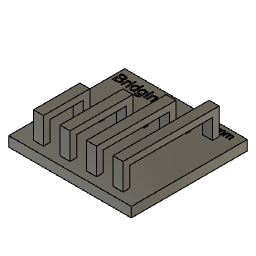
bridging (Autodesk Fusion 360 design; units mm, degrees)
Autodesk Fusion 360 part; units mm, degrees
sketch "Sketch1" plane through (0, 0, 0) normal (0, 0, 1) x (1, 0, 0)
  line L0 (0, 0) -> (37, 0)
  line L1 (37, 0) -> (37, 35)
  line L2 (37, 35) -> (0, 35)
  line L3 (0, 35) -> (0, 0)
  dimension "d1" = 35
  dimension "d2" = 37
  constraint horizontal L0
  constraint vertical L1
  constraint horizontal L2
  constraint vertical L3
  constraint coincident L0.start L3.end
  measures "d1" distance of L0.start L2.end
  measures "d2" distance of L0.start L0.end
extrude "Extrude1" add sketch "Sketch1" along normal blind 3
sketch "Sketch2" plane through (0, 0, 3) normal (0, 0, 1) x (-1, 0, 0)
  line L0 (0, -35) -> (0, 0)
  line L1 (0, 0) -> (-37, 0)
  line L2 (-37, 0) -> (-37, -35)
  line L3 (-37, -35) -> (0, -35)
  line L4 (-5, -2.5) -> (-8, -2.5)
  line L5 (-8, -2.5) -> (-8, -4.5)
  line L6 (-8, -4.5) -> (-5, -4.5)
  line L7 (-5, -4.5) -> (-5, -2.5)
  line L8 (-13, -2.5) -> (-16, -2.5)
  line L9 (-16, -2.5) -> (-16, -4.5)
  line L10 (-13, -4.5) -> (-13, -2.5)
  line L11 (-16, -4.5) -> (-13, -4.5)
  line L12 (-21, -2.5) -> (-24, -2.5)
  line L13 (-24, -2.5) -> (-24, -4.5)
  line L14 (-21, -4.5) -> (-21, -2.5)
  line L15 (-24, -4.5) -> (-21, -4.5)
  line L16 (-29, -2.5) -> (-32, -2.5)
  line L17 (-32, -2.5) -> (-32, -4.5)
  line L18 (-29, -4.5) -> (-29, -2.5)
  line L19 (-32, -4.5) -> (-29, -4.5)
  line L20 (-5, -14.5) -> (-8, -14.5)
  line L21 (-8, -14.5) -> (-8, -16.5)
  line L22 (-5, -16.5) -> (-5, -14.5)
  line L23 (-8, -16.5) -> (-5, -16.5)
  line L24 (-13, -19.5) -> (-16, -19.5)
  line L25 (-16, -19.5) -> (-16, -21.5)
  line L26 (-13, -21.5) -> (-13, -19.5)
  line L27 (-16, -21.5) -> (-13, -21.5)
  line L28 (-21, -24.5) -> (-24, -24.5)
  line L29 (-24, -24.5) -> (-24, -26.5)
  line L30 (-21, -26.5) -> (-21, -24.5)
  line L31 (-24, -26.5) -> (-21, -26.5)
  line L32 (-29, -29.5) -> (-32, -29.5)
  line L33 (-32, -29.5) -> (-32, -31.5)
  line L34 (-29, -31.5) -> (-29, -29.5)
  line L35 (-32, -31.5) -> (-29, -31.5)
  dimension "d5" = 3
  dimension "d6" = 2
  dimension "d7" = 5
  dimension "d8" = 2.5
  dimension "d9" = 3
  dimension "d10" = 2
  dimension "d11" = 3
  dimension "d12" = 2
  dimension "d13" = 3
  dimension "d14" = 2
  dimension "d15" = 3
  dimension "d16" = 2
  dimension "d17" = 3
  dimension "d18" = 2
  dimension "d19" = 3
  dimension "d20" = 2
  dimension "d21" = 3
  dimension "d22" = 2
  dimension "d23" = 10
  dimension "d24" = 15
  dimension "d25" = 20
  dimension "d26" = 25
  constraint horizontal L4
  constraint vertical L5
  constraint horizontal L6
  constraint vertical L7
  constraint horizontal L8
  constraint vertical L9
  constraint horizontal L11
  constraint vertical L10
  constraint horizontal L12
  constraint vertical L13
  constraint horizontal L15
  constraint vertical L14
  constraint horizontal L16
  constraint vertical L17
  constraint horizontal L19
  constraint vertical L18
  constraint horizontal L20
  constraint vertical L21
  constraint horizontal L23
  constraint vertical L22
  constraint horizontal L24
  constraint vertical L25
  constraint horizontal L27
  constraint vertical L26
  constraint horizontal L28
  constraint vertical L29
  constraint horizontal L31
  constraint vertical L30
  constraint horizontal L32
  constraint vertical L33
  constraint horizontal L35
  constraint vertical L34
  measures "d5" distance of L5 L7
  measures "d6" distance of L4 L6
  measures "d7" distance of L0 L7
  measures "d8" distance of L1 L4
  measures "d9" distance of L9 L10
  measures "d10" distance of L8 L11
  measures "d11" distance of L13 L14
  measures "d12" distance of L12 L15
  measures "d13" distance of L17 L18
  measures "d14" distance of L16 L19
  measures "d15" distance of L21 L22
  measures "d16" distance of L20 L23
  measures "d17" distance of L25 L26
  measures "d18" distance of L24 L27
  measures "d19" distance of L29 L30
  measures "d20" distance of L28 L31
  measures "d21" distance of L33 L34
  measures "d22" distance of L32 L35
  measures "d23" distance of L6 L20
  measures "d24" distance of L11 L24
  measures "d25" distance of L15 L28
  measures "d26" distance of L19 L32
extrude "Extrude2" add sketch "Sketch2" along normal blind 8 contours L4 L5 L6 L7 | L8 L9 L10 L11 | L12 L13 L14 L15 | L16 L17 L18 L19 | L20 L21 L22 L23 | L24 L25 L26 L27 | L28 L29 L30 L31 | L32 L33 L34 L35
sketch "Sketch3" plane through (0, 14.5, 0) normal (0, -1, 0) x (1, 0, 0)
  line L0 (5, 3) -> (8, 3)
  line L1 (8, 3) -> (8, 11)
  line L2 (8, 11) -> (5, 11)
  line L3 (5, 11) -> (5, 3)
  line L4 (5, 11) -> (8, 11)
  line L5 (8, 11) -> (8, 9)
  line L6 (8, 9) -> (5, 9)
  line L7 (5, 9) -> (5, 11)
  dimension "d29" = 2
  constraint horizontal L4
  constraint vertical L5
  constraint horizontal L6
  constraint vertical L7
  constraint coincident L2.end L3.start
  measures "d29" distance of L2.end L6.end
extrude "Extrude3" add sketch "Sketch3" along normal blind 10 contours L1 L2 L3 L4 L5 L6 L7
sketch "Sketch4" plane through (0, 19.5, 0) normal (0, -1, 0) x (1, 0, 0)
  line L0 (13, 3) -> (16, 3)
  line L1 (16, 3) -> (16, 11)
  line L2 (16, 11) -> (13, 11)
  line L3 (13, 11) -> (13, 3)
  line L4 (13, 11) -> (16, 11)
  line L5 (16, 11) -> (16, 9)
  line L6 (16, 9) -> (13, 9)
  line L7 (13, 9) -> (13, 11)
  dimension "d32" = 2
  constraint horizontal L4
  constraint vertical L5
  constraint horizontal L6
  constraint vertical L7
  constraint coincident L1 L5.end
  constraint coincident L2.end L3.start
  measures "d32" distance of L2.end L6.end
extrude "Extrude4" add sketch "Sketch4" along normal blind 15 contours L1 L2 L3 L4 L5 L6 L7
sketch "Sketch5" plane through (0, 24.5, 0) normal (0, -1, 0) x (1, 0, 0)
  line L0 (21, 3) -> (24, 3)
  line L1 (24, 3) -> (24, 11)
  line L2 (24, 11) -> (21, 11)
  line L3 (21, 11) -> (21, 3)
  line L4 (21, 11) -> (24, 11)
  line L5 (24, 11) -> (24, 9)
  line L6 (24, 9) -> (21, 9)
  line L7 (21, 9) -> (21, 11)
  dimension "d35" = 2
  constraint horizontal L4
  constraint vertical L5
  constraint horizontal L6
  constraint vertical L7
  constraint coincident L1 L5.end
  constraint coincident L2.end L3.start
  measures "d35" distance of L2.end L6.end
extrude "Extrude5" add sketch "Sketch5" along normal blind 20 contours L1 L2 L3 L4 L5 L6 L7
sketch "Sketch6" plane through (0, 29.5, 0) normal (0, -1, 0) x (1, 0, 0)
  line L0 (29, 3) -> (32, 3)
  line L1 (32, 3) -> (32, 11)
  line L2 (32, 11) -> (29, 11)
  line L3 (29, 11) -> (29, 3)
  line L4 (29, 11) -> (32, 11)
  line L5 (32, 11) -> (32, 9)
  line L6 (32, 9) -> (29, 9)
  line L7 (29, 9) -> (29, 11)
  dimension "d38" = 2
  constraint horizontal L4
  constraint vertical L5
  constraint horizontal L6
  constraint vertical L7
  constraint coincident L2.end L3.start
  measures "d38" distance of L2.end L6.end
extrude "Extrude6" add sketch "Sketch6" along normal blind 25 contours L1 L2 L3 L4 L5 L6 L7
sketch "Sketch7" plane through (0, 0, 3) normal (0, 0, 1) x (-1, 0, 0)
  line L0 (-32, -31.5) -> (-32, -29.5)
  line L1 (-32, -29.5) -> (-29, -29.5)
  line L2 (-29, -29.5) -> (-29, -31.5)
  line L3 (-29, -31.5) -> (-32, -31.5)
  line L4 (-24, -4.5) -> (-24, -2.5)
  line L5 (-24, -2.5) -> (-21, -2.5)
  line L6 (-21, -2.5) -> (-21, -4.5)
  line L7 (-21, -4.5) -> (-24, -4.5)
  line L8 (-8, -16.5) -> (-8, -14.5)
  line L9 (-8, -14.5) -> (-5, -14.5)
  line L10 (-5, -14.5) -> (-5, -16.5)
  line L11 (-5, -16.5) -> (-8, -16.5)
  line L12 (-32, -4.5) -> (-32, -2.5)
  line L13 (-32, -2.5) -> (-29, -2.5)
  line L14 (-29, -2.5) -> (-29, -4.5)
  line L15 (-29, -4.5) -> (-32, -4.5)
  line L16 (-24, -26.5) -> (-24, -24.5)
  line L17 (-24, -24.5) -> (-21, -24.5)
  line L18 (-21, -24.5) -> (-21, -26.5)
  line L19 (-21, -26.5) -> (-24, -26.5)
  line L20 (-16, -4.5) -> (-16, -2.5)
  line L21 (-16, -2.5) -> (-13, -2.5)
  line L22 (-13, -2.5) -> (-13, -4.5)
  line L23 (-13, -4.5) -> (-16, -4.5)
  line L24 (-5, -4.5) -> (-8, -4.5)
  line L25 (-8, -4.5) -> (-8, -2.5)
  line L26 (-8, -2.5) -> (-5, -2.5)
  line L27 (-5, -2.5) -> (-5, -4.5)
  line L28 (-16, -21.5) -> (-16, -19.5)
  line L29 (-16, -19.5) -> (-13, -19.5)
  line L30 (-13, -19.5) -> (-13, -21.5)
  line L31 (-13, -21.5) -> (-16, -21.5)
  line L32 (0, -35) -> (0, 0)
  line L33 (0, 0) -> (-37, 0)
  line L34 (-37, 0) -> (-37, -35)
  line L35 (-37, -35) -> (0, -35)
  line L36 (-0.8739, -29.5331) -> (-14.9892, -29.5331) construction
  line L37 (-14.9892, -29.5331) -> (-14.9892, -33.5331) construction
  line L38 (-14.9892, -33.5331) -> (-0.8739, -33.5331) construction
  line L39 (-0.8739, -33.5331) -> (-0.8739, -29.5331) construction
  text T0 "Bridging" font "Arial" height 4 align ink ink in box 0 x 0 at (-0.8839, -29.5531) x (-1, 0) y (0, -1) spacing 1 height is em
  constraint perpendicular L36 L37
  constraint parallel L36 L38
  constraint parallel L37 L39
extrude "Extrude7" cut sketch "Sketch7" against normal blind 1 text T0
sketch "Sketch8" plane through (0, 0, 3) normal (0, 0, 1) x (-1, 0, 0)
  line L0 (0, -35) -> (0, 0)
  line L1 (0, 0) -> (-37, 0)
  line L2 (-37, 0) -> (-37, -35)
  line L3 (-37, -35) -> (0, -35)
  line L4 (-16, -21.5) -> (-16, -19.5)
  line L5 (-16, -19.5) -> (-13, -19.5)
  line L6 (-13, -19.5) -> (-13, -21.5)
  line L7 (-13, -21.5) -> (-16, -21.5)
  line L8 (-5, -4.5) -> (-8, -4.5)
  line L9 (-8, -4.5) -> (-8, -2.5)
  line L10 (-8, -2.5) -> (-5, -2.5)
  line L11 (-5, -2.5) -> (-5, -4.5)
  line L12 (-16, -4.5) -> (-16, -2.5)
  line L13 (-16, -2.5) -> (-13, -2.5)
  line L14 (-13, -2.5) -> (-13, -4.5)
  line L15 (-13, -4.5) -> (-16, -4.5)
  line L16 (-24, -26.5) -> (-24, -24.5)
  line L17 (-24, -24.5) -> (-21, -24.5)
  line L18 (-21, -24.5) -> (-21, -26.5)
  line L19 (-21, -26.5) -> (-24, -26.5)
  line L20 (-32, -4.5) -> (-32, -2.5)
  line L21 (-32, -2.5) -> (-29, -2.5)
  line L22 (-29, -2.5) -> (-29, -4.5)
  line L23 (-29, -4.5) -> (-32, -4.5)
  line L24 (-8, -16.5) -> (-8, -14.5)
  line L25 (-8, -14.5) -> (-5, -14.5)
  line L26 (-5, -14.5) -> (-5, -16.5)
  line L27 (-5, -16.5) -> (-8, -16.5)
  line L28 (-24, -4.5) -> (-24, -2.5)
  line L29 (-24, -2.5) -> (-21, -2.5)
  line L30 (-21, -2.5) -> (-21, -4.5)
  line L31 (-21, -4.5) -> (-24, -4.5)
  line L32 (-32, -31.5) -> (-32, -29.5)
  line L33 (-32, -29.5) -> (-29, -29.5)
  line L34 (-29, -29.5) -> (-29, -31.5)
  line L35 (-29, -31.5) -> (-32, -31.5)
  spline S0 degree 3 poles (-2.4376, -30.4428) (-2.368, -30.4289) (-2.2156, -30.3984) (-2.0601, -30.3962) (-1.9757, -30.3949) knots 0 0 0 0 0.021277 0.046525 0.046525 0.046525 0.046525
  line L36 (-1.9757, -30.3949) -> (-0.8839, -30.3949)
  line L37 (-0.8839, -30.3949) -> (-0.8839, -33.2582)
  line L38 (-0.8839, -33.2582) -> (-1.9581, -33.2582)
  spline S1 degree 3 poles (-1.9581, -33.2582) (-2.0577, -33.2564) (-2.2376, -33.2531) (-2.4082, -33.1966) (-2.4845, -33.1713) knots 0 0 0 0 0.029645 0.05362 0.05362 0.05362 0.05362
  spline S2 degree 3 poles (-2.4845, -33.1713) (-2.5469, -33.1386) (-2.6712, -33.0734) (-2.7539, -32.9601) (-2.7951, -32.9037) knots 0 0 0 0 0.020838 0.041482 0.041482 0.041482 0.041482
  spline S3 degree 3 poles (-2.7951, -32.9037) (-2.8278, -32.8435) (-2.892, -32.7254) (-2.9023, -32.5914) (-2.9074, -32.5258) knots 0 0 0 0 0.02031 0.039825 0.039825 0.039825 0.039825
  spline S4 degree 3 poles (-2.9074, -32.5258) (-2.9031, -32.4653) (-2.8944, -32.343) (-2.8368, -32.2347) (-2.8078, -32.1801) knots 0 0 0 0 0.017995 0.036334 0.036334 0.036334 0.036334
  spline S5 degree 3 poles (-2.8078, -32.1801) (-2.769, -32.128) (-2.6878, -32.0191) (-2.569, -31.9529) (-2.507, -31.9184) knots 0 0 0 0 0.019257 0.040275 0.040275 0.040275 0.040275
  spline S6 degree 3 poles (-2.507, -31.9184) (-2.5874, -31.8899) (-2.7417, -31.8354) (-2.8531, -31.7158) (-2.9064, -31.6586) knots 0 0 0 0 0.025178 0.048277 0.048277 0.048277 0.048277
  spline S7 degree 3 poles (-2.9064, -31.6586) (-2.9471, -31.5938) (-3.0304, -31.4612) (-3.0407, -31.3049) (-3.046, -31.225) knots 0 0 0 0 0.022594 0.046193 0.046193 0.046193 0.046193
  spline S8 degree 3 poles (-3.046, -31.225) (-3.0427, -31.1595) (-3.036, -31.0299) (-2.9859, -30.9102) (-2.9611, -30.851) knots 0 0 0 0 0.019525 0.038613 0.038613 0.038613 0.038613
  spline S9 degree 3 poles (-2.9611, -30.851) (-2.9323, -30.7976) (-2.8778, -30.6964) (-2.7918, -30.6204) (-2.7511, -30.5844) knots 0 0 0 0 0.018014 0.034173 0.034173 0.034173 0.034173
  spline S10 degree 3 poles (-2.7511, -30.5844) (-2.7052, -30.5547) (-2.608, -30.4917) (-2.4965, -30.4597) (-2.4376, -30.4428) knots 0 0 0 0 0.016314 0.034565 0.034565 0.034565 0.034565
  line L39 (-5.2082, -33.2582) -> (-5.2082, -32.8539)
  line L40 (-5.2082, -32.8539) -> (-4.8566, -32.8539)
  line L41 (-4.8566, -32.8539) -> (-4.8566, -33.2582)
  line L42 (-4.8566, -33.2582) -> (-5.2082, -33.2582)
  line L43 (-7.4152, -33.2582) -> (-7.4152, -30.3949)
  line L44 (-7.4152, -30.3949) -> (-7.089, -30.3949)
  line L45 (-7.089, -30.3949) -> (-7.089, -30.6567)
  spline S11 degree 3 poles (-7.089, -30.6567) (-7.0147, -30.5667) (-6.864, -30.3842) (-6.6284, -30.3602) (-6.5089, -30.3481) knots 0 0 0 0 0.033606 0.068121 0.068121 0.068121 0.068121
  spline S12 degree 3 poles (-6.5089, -30.3481) (-6.4279, -30.3538) (-6.2656, -30.3652) (-6.1238, -30.4449) (-6.0529, -30.4848) knots 0 0 0 0 0.024048 0.048141 0.048141 0.048141 0.048141
  spline S13 degree 3 poles (-6.0529, -30.4848) (-5.9871, -30.5357) (-5.8524, -30.6399) (-5.7718, -30.79) (-5.7306, -30.8666) knots 0 0 0 0 0.024678 0.050464 0.050464 0.050464 0.050464
  spline S14 degree 3 poles (-5.7306, -30.8666) (-5.6973, -30.9534) (-5.6278, -31.1347) (-5.6203, -31.3289) (-5.6164, -31.4301) knots 0 0 0 0 0.027702 0.057842 0.057842 0.057842 0.057842
  spline S15 degree 3 poles (-5.6164, -31.4301) (-5.6201, -31.5297) (-5.6273, -31.7227) (-5.6897, -31.9053) (-5.7199, -31.9936) knots 0 0 0 0 0.029727 0.057565 0.057565 0.057565 0.057565
  spline S16 degree 3 poles (-5.7199, -31.9936) (-5.7577, -32.0723) (-5.8314, -32.2256) (-5.9653, -32.3303) (-6.0304, -32.3813) knots 0 0 0 0 0.025816 0.050272 0.050272 0.050272 0.050272
  spline S17 degree 3 poles (-6.0304, -32.3813) (-6.1019, -32.4206) (-6.2461, -32.4999) (-6.4104, -32.5106) (-6.4933, -32.516) knots 0 0 0 0 0.024142 0.048739 0.048739 0.048739 0.048739
  spline S18 degree 3 poles (-6.4933, -32.516) (-6.5533, -32.5132) (-6.6696, -32.5076) (-6.7758, -32.46) (-6.8273, -32.4369) knots 0 0 0 0 0.017835 0.034594 0.034594 0.034594 0.034594
  spline S19 degree 3 poles (-6.8273, -32.4369) (-6.8736, -32.4089) (-6.9648, -32.3538) (-7.0323, -32.2714) (-7.0656, -32.2309) knots 0 0 0 0 0.016103 0.031707 0.031707 0.031707 0.031707
  line L46 (-7.0656, -32.2309) -> (-7.0656, -33.2582)
  line L47 (-7.0656, -33.2582) -> (-7.4152, -33.2582)
  spline S20 degree 3 poles (-8.7238, -29.5531) (-8.6093, -29.5579) (-8.3958, -29.5666) (-8.2102, -29.6715) (-8.1242, -29.7201) knots 0 0 0 0 0.033804 0.063038 0.063038 0.063038 0.063038
  spline S21 degree 3 poles (-8.1242, -29.7201) (-8.0579, -29.7855) (-7.9184, -29.9231) (-7.9086, -30.1197) (-7.9035, -30.2231) knots 0 0 0 0 0.026923 0.056737 0.056737 0.056737 0.056737
  line L48 (-7.9035, -30.2231) -> (-8.2453, -30.1723)
  spline S22 degree 3 poles (-8.2453, -30.1723) (-8.2542, -30.1243) (-8.2708, -30.035) (-8.3348, -29.9713) (-8.3644, -29.9418) knots 0 0 0 0 0.01426 0.026495 0.026495 0.026495 0.026495
  spline S23 degree 3 poles (-8.3644, -29.9418) (-8.4148, -29.9134) (-8.5254, -29.8511) (-8.6526, -29.8466) (-8.7218, -29.8442) knots 0 0 0 0 0.017124 0.037534 0.037534 0.037534 0.037534
  spline S24 degree 3 poles (-8.7218, -29.8442) (-8.7956, -29.8462) (-8.9292, -29.85) (-9.0463, -29.9134) (-9.0988, -29.9418) knots 0 0 0 0 0.021768 0.039424 0.039424 0.039424 0.039424
  spline S25 degree 3 poles (-9.0988, -29.9418) (-9.1397, -29.9784) (-9.2237, -30.0535) (-9.2599, -30.1604) (-9.2785, -30.2153) knots 0 0 0 0 0.016164 0.033219 0.033219 0.033219 0.033219
  spline S26 degree 3 poles (-9.2785, -30.2153) (-9.2862, -30.2707) (-9.307, -30.4202) (-9.3051, -30.5713) (-9.3039, -30.6664) knots 0 0 0 0 0.01677 0.045242 0.045242 0.045242 0.045242
  spline S27 degree 3 poles (-9.3039, -30.6664) (-9.2229, -30.5872) (-9.0626, -30.4305) (-8.8399, -30.4067) (-8.7296, -30.3949) knots 0 0 0 0 0.032929 0.065194 0.065194 0.065194 0.065194
  spline S28 degree 3 poles (-8.7296, -30.3949) (-8.5963, -30.4062) (-8.3372, -30.4282) (-8.1557, -30.6136) (-8.0675, -30.7035) knots 0 0 0 0 0.038716 0.075253 0.075253 0.075253 0.075253
  spline S29 degree 3 poles (-8.0675, -30.7035) (-7.9992, -30.8135) (-7.8584, -31.0401) (-7.8417, -31.3066) (-7.8332, -31.4438) knots 0 0 0 0 0.038218 0.078732 0.078732 0.078732 0.078732
  spline S30 degree 3 poles (-7.8332, -31.4438) (-7.8372, -31.5399) (-7.8452, -31.728) (-7.9092, -31.905) (-7.9406, -31.9916) knots 0 0 0 0 0.028666 0.05612 0.05612 0.05612 0.05612
  spline S31 degree 3 poles (-7.9406, -31.9916) (-7.9794, -32.0698) (-8.055, -32.222) (-8.1876, -32.3279) (-8.2521, -32.3793) knots 0 0 0 0 0.025842 0.050275 0.050275 0.050275 0.050275
  spline S32 degree 3 poles (-8.2521, -32.3793) (-8.3244, -32.4192) (-8.4736, -32.5014) (-8.6439, -32.5111) (-8.7316, -32.516) knots 0 0 0 0 0.024447 0.050429 0.050429 0.050429 0.050429
  spline S33 degree 3 poles (-8.7316, -32.516) (-8.849, -32.5032) (-9.0864, -32.4771) (-9.2529, -32.3057) (-9.3371, -32.2192) knots 0 0 0 0 0.034309 0.069344 0.069344 0.069344 0.069344
  line L49 (-9.3371, -32.2192) -> (-9.3371, -32.4692)
  line L50 (-9.3371, -32.4692) -> (-9.6613, -32.4692)
  line L51 (-9.6613, -32.4692) -> (-9.6613, -30.6762)
  spline S34 degree 3 poles (-9.6613, -30.6762) (-9.6614, -30.5369) (-9.6615, -30.3026) (-9.5912, -30.0799) (-9.5626, -29.9897) knots 0 0 0 0 0.041455 0.069711 0.069711 0.069711 0.069711
  spline S35 degree 3 poles (-9.5626, -29.9897) (-9.5242, -29.9254) (-9.4457, -29.7941) (-9.3163, -29.7122) (-9.2501, -29.6703) knots 0 0 0 0 0.022129 0.045239 0.045239 0.045239 0.045239
  spline S36 degree 3 poles (-9.2501, -29.6703) (-9.1718, -29.6362) (-9.0041, -29.5632) (-8.8212, -29.5566) (-8.7238, -29.5531) knots 0 0 0 0 0.02542 0.054353 0.054353 0.054353 0.054353
  line L52 (-10.546, -32.4692) -> (-10.546, -30.3949)
  line L53 (-10.546, -30.3949) -> (-10.1945, -30.3949)
  line L54 (-10.1945, -30.3949) -> (-10.1945, -32.4692)
  line L55 (-10.1945, -32.4692) -> (-10.546, -32.4692)
  line L56 (-11.4328, -31.5278) -> (-11.4328, -30.3949)
  line L57 (-11.4328, -30.3949) -> (-11.0812, -30.3949)
  line L58 (-11.0812, -30.3949) -> (-11.0812, -32.4692)
  line L59 (-11.0812, -32.4692) -> (-11.3976, -32.4692)
  line L60 (-11.3976, -32.4692) -> (-11.3976, -32.1742)
  spline S37 degree 3 poles (-11.3976, -32.1742) (-11.4833, -32.2739) (-11.6571, -32.4762) (-11.9229, -32.5026) (-12.0578, -32.516) knots 0 0 0 0 0.037911 0.076943 0.076943 0.076943 0.076943
  spline S38 degree 3 poles (-12.0578, -32.516) (-12.1183, -32.5135) (-12.2367, -32.5086) (-12.3481, -32.4683) (-12.4025, -32.4487) knots 0 0 0 0 0.018072 0.035309 0.035309 0.035309 0.035309
  spline S39 degree 3 poles (-12.4025, -32.4487) (-12.4506, -32.4257) (-12.5412, -32.3826) (-12.607, -32.3072) (-12.6378, -32.2719) knots 0 0 0 0 0.015798 0.029713 0.029713 0.029713 0.029713
  spline S40 degree 3 poles (-12.6378, -32.2719) (-12.6621, -32.2329) (-12.7123, -32.1522) (-12.7353, -32.0599) (-12.7472, -32.0121) knots 0 0 0 0 0.013682 0.02834 0.02834 0.02834 0.02834
  spline S41 degree 3 poles (-12.7472, -32.0121) (-12.7528, -31.9674) (-12.7671, -31.854) (-12.7669, -31.7396) (-12.7667, -31.6703) knots 0 0 0 0 0.013507 0.034265 0.034265 0.034265 0.034265
  line L61 (-12.7667, -31.6703) -> (-12.7667, -30.3949)
  line L62 (-12.7667, -30.3949) -> (-12.4152, -30.3949)
  line L63 (-12.4152, -30.3949) -> (-12.4152, -31.6567)
  spline S42 degree 3 poles (-12.4152, -31.6567) (-12.4148, -31.7197) (-12.4143, -31.8286) (-12.3861, -31.9337) (-12.3742, -31.978) knots 0 0 0 0 0.018802 0.032507 0.032507 0.032507 0.032507
  spline S43 degree 3 poles (-12.3742, -31.978) (-12.3575, -32.0118) (-12.3236, -32.0809) (-12.2607, -32.1253) (-12.2287, -32.1479) knots 0 0 0 0 0.011133 0.022693 0.022693 0.022693 0.022693
  spline S44 degree 3 poles (-12.2287, -32.1479) (-12.1915, -32.1664) (-12.1144, -32.2048) (-12.0282, -32.2091) (-11.9835, -32.2114) knots 0 0 0 0 0.01231 0.025565 0.025565 0.025565 0.025565
  spline S45 degree 3 poles (-11.9835, -32.2114) (-11.9115, -32.2057) (-11.7689, -32.1944) (-11.6531, -32.1104) (-11.5958, -32.0688) knots 0 0 0 0 0.021224 0.042029 0.042029 0.042029 0.042029
  spline S46 degree 3 poles (-11.5958, -32.0688) (-11.5486, -32.0021) (-11.4351, -31.8419) (-11.4336, -31.6436) (-11.4328, -31.5278) knots 0 0 0 0 0.024004 0.057699 0.057699 0.057699 0.057699
  line L64 (-10.546, -33.2582) -> (-10.546, -32.8539)
  line L65 (-10.546, -32.8539) -> (-10.1945, -32.8539)
  line L66 (-10.1945, -32.8539) -> (-10.1945, -33.2582)
  line L67 (-10.1945, -33.2582) -> (-10.546, -33.2582)
  spline S47 degree 3 poles (-14.0617, -29.5531) (-13.9472, -29.5579) (-13.7336, -29.5666) (-13.5481, -29.6715) (-13.4621, -29.7201) knots 0 0 0 0 0.033804 0.063038 0.063038 0.063038 0.063038
  spline S48 degree 3 poles (-13.4621, -29.7201) (-13.3958, -29.7855) (-13.2563, -29.9231) (-13.2465, -30.1197) (-13.2414, -30.2231) knots 0 0 0 0 0.026923 0.056737 0.056737 0.056737 0.056737
  line L68 (-13.2414, -30.2231) -> (-13.5831, -30.1723)
  spline S49 degree 3 poles (-13.5831, -30.1723) (-13.5921, -30.1243) (-13.6087, -30.035) (-13.6727, -29.9713) (-13.7023, -29.9418) knots 0 0 0 0 0.01426 0.026495 0.026495 0.026495 0.026495
  spline S50 degree 3 poles (-13.7023, -29.9418) (-13.7527, -29.9134) (-13.8633, -29.8511) (-13.9905, -29.8466) (-14.0597, -29.8442) knots 0 0 0 0 0.017124 0.037534 0.037534 0.037534 0.037534
  spline S51 degree 3 poles (-14.0597, -29.8442) (-14.1335, -29.8462) (-14.2671, -29.85) (-14.3842, -29.9134) (-14.4367, -29.9418) knots 0 0 0 0 0.021768 0.039424 0.039424 0.039424 0.039424
  spline S52 degree 3 poles (-14.4367, -29.9418) (-14.4775, -29.9784) (-14.5616, -30.0535) (-14.5978, -30.1604) (-14.6164, -30.2153) knots 0 0 0 0 0.016164 0.033219 0.033219 0.033219 0.033219
  spline S53 degree 3 poles (-14.6164, -30.2153) (-14.6241, -30.2707) (-14.6449, -30.4202) (-14.643, -30.5713) (-14.6417, -30.6664) knots 0 0 0 0 0.01677 0.045242 0.045242 0.045242 0.045242
  spline S54 degree 3 poles (-14.6417, -30.6664) (-14.5608, -30.5872) (-14.4005, -30.4305) (-14.1778, -30.4067) (-14.0675, -30.3949) knots 0 0 0 0 0.032929 0.065194 0.065194 0.065194 0.065194
  spline S55 degree 3 poles (-14.0675, -30.3949) (-13.9342, -30.4062) (-13.6751, -30.4282) (-13.4936, -30.6136) (-13.4054, -30.7035) knots 0 0 0 0 0.038716 0.075253 0.075253 0.075253 0.075253
  spline S56 degree 3 poles (-13.4054, -30.7035) (-13.3371, -30.8135) (-13.1963, -31.0401) (-13.1796, -31.3066) (-13.171, -31.4438) knots 0 0 0 0 0.038218 0.078732 0.078732 0.078732 0.078732
  spline S57 degree 3 poles (-13.171, -31.4438) (-13.1751, -31.5399) (-13.1831, -31.728) (-13.2471, -31.905) (-13.2785, -31.9916) knots 0 0 0 0 0.028666 0.05612 0.05612 0.05612 0.05612
  spline S58 degree 3 poles (-13.2785, -31.9916) (-13.3173, -32.0698) (-13.3928, -32.222) (-13.5255, -32.3279) (-13.59, -32.3793) knots 0 0 0 0 0.025842 0.050275 0.050275 0.050275 0.050275
  spline S59 degree 3 poles (-13.59, -32.3793) (-13.6623, -32.4192) (-13.8115, -32.5014) (-13.9818, -32.5111) (-14.0695, -32.516) knots 0 0 0 0 0.024447 0.050429 0.050429 0.050429 0.050429
  spline S60 degree 3 poles (-14.0695, -32.516) (-14.1869, -32.5032) (-14.4243, -32.4771) (-14.5908, -32.3057) (-14.6749, -32.2192) knots 0 0 0 0 0.034309 0.069344 0.069344 0.069344 0.069344
  line L69 (-14.6749, -32.2192) -> (-14.6749, -32.4692)
  line L70 (-14.6749, -32.4692) -> (-14.9992, -32.4692)
  line L71 (-14.9992, -32.4692) -> (-14.9992, -30.6762)
  spline S61 degree 3 poles (-14.9992, -30.6762) (-14.9993, -30.5369) (-14.9994, -30.3026) (-14.9291, -30.0799) (-14.9005, -29.9897) knots 0 0 0 0 0.041455 0.069711 0.069711 0.069711 0.069711
  spline S62 degree 3 poles (-14.9005, -29.9897) (-14.8621, -29.9254) (-14.7836, -29.7941) (-14.6541, -29.7122) (-14.588, -29.6703) knots 0 0 0 0 0.022129 0.045239 0.045239 0.045239 0.045239
  spline S63 degree 3 poles (-14.588, -29.6703) (-14.5096, -29.6362) (-14.342, -29.5632) (-14.1591, -29.5566) (-14.0617, -29.5531) knots 0 0 0 0 0.02542 0.054353 0.054353 0.054353 0.054353
  line L72 (-5.2082, -32.4692) -> (-5.2082, -30.3949)
  line L73 (-5.2082, -30.3949) -> (-4.8566, -30.3949)
  line L74 (-4.8566, -30.3949) -> (-4.8566, -32.4692)
  line L75 (-4.8566, -32.4692) -> (-5.2082, -32.4692)
  line L76 (-3.8703, -31.4809) -> (-3.8703, -30.3949)
  line L77 (-3.8703, -30.3949) -> (-3.5187, -30.3949)
  line L78 (-3.5187, -30.3949) -> (-3.5187, -32.4692)
  line L79 (-3.5187, -32.4692) -> (-3.8351, -32.4692)
  line L80 (-3.8351, -32.4692) -> (-3.8351, -32.1547)
  spline S64 degree 3 poles (-3.8351, -32.1547) (-3.8703, -32.2186) (-3.9303, -32.3273) (-4.0213, -32.4112) (-4.0587, -32.4457) knots 0 0 0 0 0.0217 0.036909 0.036909 0.036909 0.036909
  spline S65 degree 3 poles (-4.0587, -32.4457) (-4.0937, -32.4662) (-4.1635, -32.5071) (-4.2441, -32.5131) (-4.2843, -32.516) knots 0 0 0 0 0.011989 0.023911 0.023911 0.023911 0.023911
  spline S66 degree 3 poles (-4.2843, -32.516) (-4.3452, -32.5104) (-4.4736, -32.4986) (-4.5864, -32.4358) (-4.6457, -32.4028) knots 0 0 0 0 0.018142 0.038239 0.038239 0.038239 0.038239
  line L81 (-4.6457, -32.4028) -> (-4.5246, -32.0766)
  spline S67 degree 3 poles (-4.5246, -32.0766) (-4.4825, -32.0988) (-4.4016, -32.1415) (-4.3105, -32.1491) (-4.2667, -32.1528) knots 0 0 0 0 0.0141 0.02713 0.02713 0.02713 0.02713
  spline S68 degree 3 poles (-4.2667, -32.1528) (-4.2293, -32.1499) (-4.1545, -32.1441) (-4.0913, -32.1036) (-4.0597, -32.0834) knots 0 0 0 0 0.011074 0.022138 0.022138 0.022138 0.022138
  spline S69 degree 3 poles (-4.0597, -32.0834) (-4.0311, -32.0575) (-3.9721, -32.0039) (-3.9436, -31.9294) (-3.9289, -31.891) knots 0 0 0 0 0.011415 0.023558 0.023558 0.023558 0.023558
  spline S70 degree 3 poles (-3.9289, -31.891) (-3.9118, -31.826) (-3.8765, -31.6915) (-3.8724, -31.5526) (-3.8703, -31.4809) knots 0 0 0 0 0.020115 0.041552 0.041552 0.041552 0.041552
  line L82 (-2.4238, -17.2714) -> (-10.2387, -17.2714) construction
  line L83 (-10.2387, -17.2714) -> (-10.2387, -20.2714) construction
  line L84 (-10.2387, -20.2714) -> (-2.4238, -20.2714) construction
  line L85 (-2.4238, -20.2714) -> (-2.4238, -17.2714) construction
  line L86 (-10.619, -22.2917) -> (-18.4339, -22.2917) construction
  line L87 (-18.4339, -22.2917) -> (-18.4339, -25.2917) construction
  line L88 (-18.4339, -25.2917) -> (-10.619, -25.2917) construction
  line L89 (-10.619, -25.2917) -> (-10.619, -22.2917) construction
  line L90 (-18.1891, -27.1804) -> (-26.2429, -27.1804) construction
  line L91 (-26.2429, -27.1804) -> (-26.2429, -30.1804) construction
  line L92 (-26.2429, -30.1804) -> (-18.1891, -30.1804) construction
  line L93 (-18.1891, -30.1804) -> (-18.1891, -27.1804) construction
  line L94 (-26.2593, -32.2242) -> (-34.313, -32.2242) construction
  line L95 (-34.313, -32.2242) -> (-34.313, -35.2242) construction
  line L96 (-34.313, -35.2242) -> (-26.2593, -35.2242) construction
  line L97 (-26.2593, -35.2242) -> (-26.2593, -32.2242) construction
  text T0 "10mm" font "Arial" height 3 align ink ink in box 0 x 0 at (-2.4338, -17.2914) x (-1, 0) y (0, -1) spacing 1 height is em
  text T1 "15mm" font "Arial" height 3 align ink ink in box 0 x 0 at (-10.629, -22.3117) x (-1, 0) y (0, -1) spacing 1 height is em
  text T2 "20mm" font "Arial" height 3 align ink ink in box 0 x 0 at (-18.1991, -27.2004) x (-1, 0) y (0, -1) spacing 1 height is em
  text T3 "25mm" font "Arial" height 3 align ink ink in box 0 x 0 at (-26.2693, -32.2442) x (-1, 0) y (0, -1) spacing 1 height is em
  constraint perpendicular L82 L83
  constraint parallel L82 L84
  constraint parallel L83 L85
  constraint perpendicular L86 L87
  constraint parallel L86 L88
  constraint parallel L87 L89
  constraint perpendicular L90 L91
  constraint parallel L90 L92
  constraint parallel L91 L93
  constraint perpendicular L94 L95
  constraint parallel L94 L96
  constraint parallel L95 L97
extrude "Extrude8" cut sketch "Sketch8" against normal blind 1 text T0 T1 T2 T3
